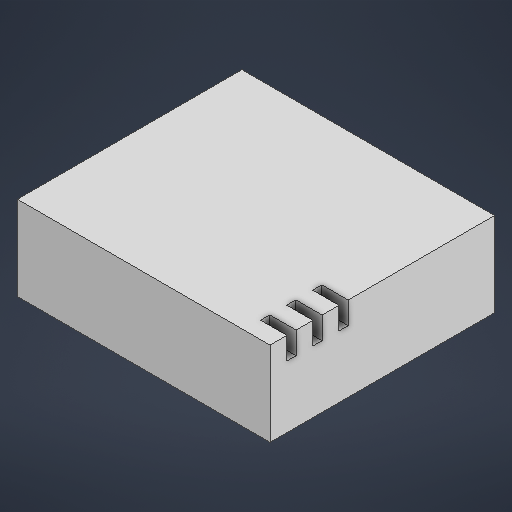
# Autodesk Inventor part: S009_3.7V_Li-ion_Battery_900mAh_3.33Wh
Saved by Autodesk Inventor 2026.2 (Build 302298000, 298)
## iProperties
Created: 2026-02-06
Part Number: S009_3.7V_Li-ion_Battery_900mAh_3.33Wh
Material: 一般
Document SubType Name: Modeling
Designer: Willy
Density: 1 g/cm^3
Appearance: 預設
Author: Willy
Autodesk Inventor part; units mm, degrees
ref_plane "YZ Plane" through (0, 0, 0) normal (1, 0, 0) x (0, 1, 0)
ref_plane "XZ Plane" through (0, 0, 0) normal (0, 1, 0) x (-1, 0, 0)
ref_plane "XY Plane" through (0, 0, 0) normal (0, 0, 1) x (1, 0, 0)
sketch "草圖1" plane through (0, 0, 0) normal (0, 1, 0) x (-1, 0, 0)
  line L0 (-16.5, 14.66) -> (16.5, 14.66)
  line L1 (16.5, 14.66) -> (16.5, -14.66)
  line L2 (16.5, -14.66) -> (-16.5, -14.66)
  line L3 (-16.5, -14.66) -> (-16.5, 14.66)
  line L4 (-16.5, 14.66) -> (16.5, -14.66) construction
  line L5 (16.5, 14.66) -> (-16.5, -14.66) construction
  point P0 (0, 0)
  dimension "d0" = 29.32
  dimension "d1" = 33
  constraints: 12 end point, 2 midpoint, 2 parallel, 1 horizontal, 1 perpendicular
  measures "d0" distance of L0.end L1.end
  measures "d1" distance of L1.end L2.end
extrude "擠出1" add sketch "草圖1" along normal mid plane 11
sketch "草圖2" plane through (0, 5.5, 0) normal (0, 1, 0) x (1, 0, 0)
  line L0 (16.5, -14.66) -> (16.5, 14.66) projected
  line L1 (16.5, -12.46) -> (13.06, -12.46)
  line L2 (13.06, -12.46) -> (13.06, -11.26)
  line L3 (13.06, -11.26) -> (16.5, -11.26)
  line L4 (16.5, -11.26) -> (16.5, -12.46)
  line L5 (-16.5, -14.66) -> (16.5, -14.66) projected
  line L6 (16.5, -9.06) -> (13.06, -9.06)
  line L7 (13.06, -9.06) -> (13.06, -7.86)
  line L8 (13.06, -7.86) -> (16.5, -7.86)
  line L9 (16.5, -7.86) -> (16.5, -9.06)
  line L10 (16.5, -5.66) -> (13.06, -5.66)
  line L11 (13.06, -5.66) -> (13.06, -4.46)
  line L12 (13.06, -4.46) -> (16.5, -4.46)
  line L13 (16.5, -4.46) -> (16.5, -5.66)
  point P0 (0, 0)
  point P1 (16.5, -5.66)
  point P2 (16.5, -4.46)
  dimension "d4" = 1.2
  dimension "d5" = 3.44
  dimension "d6" = 2.2
  dimension "d9" = 3.4
  constraints: 24 end point, 2 parallel, 1 horizontal, 1 perpendicular, 1 point on line, 1 vertical, 16 other
  measures "d4" distance of L1.end L2.end
  measures "d5" distance of L2.end L3.end
  measures "d6" distance between parallel lines of L5 L1
  measures "d9" distance of L1.start L6.start
extrude "擠出2" cut sketch "草圖2" against normal blind 2.9
